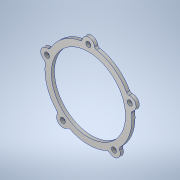
# Autodesk Inventor part: 조인트4베어링관절2
Saved by Autodesk Inventor 2020 (Build 240168000, 168)
## iProperties
Created: 2021-07-16
Part Number: 조인트4베어링관절2
Material: 알루미늄 6061
Document SubType Name: Modeling
Designer: user
Density: 2.7 g/cm^3
Appearance: 알루미늄 - 평지
Mass: 4.02174 g
Surface Area: 22.7664 cm^2
Volume: 1.48953 cm^3
Author: user
Autodesk Inventor part; units mm, degrees
ref_plane "YZ Plane" through (0, 0, 0) normal (1, 0, 0) x (0, 1, 0)
ref_plane "XZ Plane" through (0, 0, 0) normal (0, 1, 0) x (-1, 0, 0)
ref_plane "XY Plane" through (0, 0, 0) normal (0, 0, 1) x (1, 0, 0)
sketch "스케치1" plane through (0, 0, 0) normal (0, 0, 1) x (1, 0, 0)
  circle A0 centre (0, 0) radius 23.535
  circle A1 centre (0, 0) radius 27.6
  line L0 (0, 0) -> (0, 27.6)
  circle A2 centre (0, 27.6) radius 4
  circle A3 centre (-26.2492, 8.5289) radius 4
  circle A4 centre (-16.2229, -22.3289) radius 4
  circle A5 centre (16.2229, -22.3289) radius 4
  circle A6 centre (26.2492, 8.5289) radius 4
  dimension "d1" = 55.2
  dimension "d0" = 47.07
  dimension "d2" = 8
  dimension "d5" = 360
  constraints: 6 centre point, 3 coincident, 2 end point, 1 vertical, 1 vertical alignment, 13 other
  measures "d0" diameter of A0
  measures "d2" diameter of A2
extrude "돌출1" add sketch "스케치1" along normal blind 2
sketch "스케치2" plane through (0, 0, 2) normal (0, 0, 1) x (1, 0, 0)
  circle A0 centre (0, 0) radius 23.535 projected
  arc A1 (24.7407, 12.2335) -> (3.9895, 27.3101) centre (0, 0) ccw projected
  arc A2 (3.9895, 27.3101) -> (-3.9895, 27.3101) centre (0, 27.6) ccw projected
  arc A3 (-3.9895, 27.3101) -> (-24.7407, 12.2335) centre (0, 0) ccw projected
  arc A4 (-24.7407, 12.2335) -> (-27.2063, 4.6451) centre (-26.2492, 8.5289) ccw projected
  arc A5 (-27.2063, 4.6451) -> (-19.2801, -19.7494) centre (0, 0) ccw projected
  arc A6 (-19.2801, -19.7494) -> (-12.8249, -24.4393) centre (-16.2229, -22.3289) ccw projected
  arc A7 (-12.8249, -24.4393) -> (12.8249, -24.4393) centre (0, 0) ccw projected
  arc A8 (12.8249, -24.4393) -> (19.2801, -19.7494) centre (16.2229, -22.3289) ccw projected
  arc A9 (19.2801, -19.7494) -> (27.2063, 4.6451) centre (0, 0) ccw projected
  arc A10 (27.2063, 4.6451) -> (24.7407, 12.2335) centre (26.2492, 8.5289) ccw projected
  circle A11 centre (-26.2492, 8.5289) radius 1.6
  circle A12 centre (-16.2229, -22.3289) radius 1.6
  circle A13 centre (16.2229, -22.3289) radius 1.6
  circle A14 centre (26.2492, 8.5289) radius 1.6
  circle A15 centre (0, 27.6) radius 1.6
  dimension "d9" = 3.2
  dimension "d10" = 3.2
  dimension "d11" = 3.2
  dimension "d12" = 3.2
  dimension "d13" = 3.2
  constraints: 5 centre point, 5 coincident
  measures "d9" diameter of A11
  measures "d10" diameter of A12
  measures "d11" diameter of A13
  measures "d12" diameter of A14
  measures "d13" diameter of A15
extrude "돌출2" cut sketch "스케치2" against normal up to surface (2 mm away) contours A11 | A12 | A13 | A14 | A15
fillet "모깎기1" radius 1.5 10 edges at (-19.2801, -19.7494, 1) (-12.8249, -24.4393, 1) (19.2801, -19.7494, 1) (12.8249, -24.4393, 1) (24.7407, 12.2335, 1) (27.2063, 4.6451, 1) (3.9895, 27.3101, 1) (-3.9895, 27.3101, 1) (-24.7407, 12.2335, 1) (-27.2063, 4.6451, 1)
